Motor to Extrusion Adaptor_v5 (Autodesk Fusion 360 design; units mm, degrees)
Autodesk Fusion 360 part; units mm, degrees
sketch "Sketch1" plane through (0, 0, 0) normal (0, 0, 1) x (1, 0, 0)
  line L0 (0, 0) -> (84, 0)
  line L1 (84, 0) -> (84, 60)
  line L2 (84, 60) -> (0, 60)
  line L3 (0, 60) -> (0, 0)
  line L4 (5, 60) -> (5, 0) construction
  line L5 (79, 60) -> (79, 0) construction
  line L6 (5, 50) -> (79, 50) construction
  line L7 (5, 10) -> (79, 10) construction
  line L8 (7.75, 50) -> (7.75, 10) construction
  line L9 (76.25, 50) -> (76.25, 10) construction
  line L10 (5, 55) -> (79, 55) construction
  line L11 (5, 5) -> (79, 5) construction
  line L12 (7.75, 10) -> (7.75, 5) construction
  line L13 (7.75, 50) -> (7.75, 55) construction
  line L14 (76.25, 50) -> (76.25, 55) construction
  line L15 (76.25, 10) -> (76.25, 5) construction
  line L16 (7.75, 15) -> (76.25, 15) construction
  line L17 (7.75, 45) -> (76.25, 45) construction
  line L18 (5, 55) -> (5, 45)
  arc A0 (5, 45) -> (10.5, 45) centre (7.75, 45) ccw
  line L19 (10.5, 45) -> (10.5, 55)
  arc A1 (10.5, 55) -> (5, 55) centre (7.75, 55) ccw
  line L20 (7.75, 55) -> (7.75, 45) construction
  line L21 (10.5, 5) -> (10.5, 15)
  arc A2 (10.5, 15) -> (5, 15) centre (7.75, 15) ccw
  line L22 (5, 15) -> (5, 5)
  arc A3 (5, 5) -> (10.5, 5) centre (7.75, 5) ccw
  line L23 (7.75, 5) -> (7.75, 15) construction
  line L24 (73.5, 55) -> (73.5, 45)
  arc A4 (73.5, 45) -> (79, 45) centre (76.25, 45) ccw
  line L25 (79, 45) -> (79, 55)
  arc A5 (79, 55) -> (73.5, 55) centre (76.25, 55) ccw
  line L26 (76.25, 55) -> (76.25, 45) construction
  line L27 (73.5, 15) -> (73.5, 5)
  arc A6 (73.5, 5) -> (79, 5) centre (76.25, 5) ccw
  line L28 (79, 5) -> (79, 15)
  arc A7 (79, 15) -> (73.5, 15) centre (76.25, 15) ccw
  line L29 (76.25, 15) -> (76.25, 5) construction
  line L30 (15.5, 55) -> (68.5, 55)
  line L31 (68.5, 55) -> (68.5, 5)
  line L32 (68.5, 5) -> (15.5, 5)
  line L33 (15.5, 5) -> (15.5, 55)
  line L34 (15.5, 55) -> (68.5, 5) construction
  line L35 (68.5, 55) -> (15.5, 5) construction
  line L36 (68.5, 55) -> (68.5, 5) construction
  line L37 (15.5, 55) -> (15.5, 5) construction
  line L38 (50, 15) -> (50, 45) construction
  line L39 (34, 15) -> (34, 45) construction
  line L40 (31.9215, 18.6) -> (29.8431, 15)
  line L41 (29.8431, 15) -> (31.9215, 11.4)
  line L42 (31.9215, 11.4) -> (36.0785, 11.4)
  line L43 (36.0785, 11.4) -> (38.1569, 15)
  line L44 (38.1569, 15) -> (36.0785, 18.6)
  line L45 (36.0785, 18.6) -> (31.9215, 18.6)
  line L46 (36.0785, 41.4) -> (38.1569, 45)
  line L47 (38.1569, 45) -> (36.0785, 48.6)
  line L48 (36.0785, 48.6) -> (31.9215, 48.6)
  line L49 (31.9215, 48.6) -> (29.8431, 45)
  line L50 (29.8431, 45) -> (31.9215, 41.4)
  line L51 (31.9215, 41.4) -> (36.0785, 41.4)
  line L52 (52.0785, 41.4) -> (54.1569, 45)
  line L53 (54.1569, 45) -> (52.0785, 48.6)
  line L54 (52.0785, 48.6) -> (47.9215, 48.6)
  line L55 (47.9215, 48.6) -> (45.8431, 45)
  line L56 (45.8431, 45) -> (47.9215, 41.4)
  line L57 (47.9215, 41.4) -> (52.0785, 41.4)
  line L58 (47.9215, 18.6) -> (45.8431, 15)
  line L59 (45.8431, 15) -> (47.9215, 11.4)
  line L60 (47.9215, 11.4) -> (52.0785, 11.4)
  line L61 (52.0785, 11.4) -> (54.1569, 15)
  line L62 (54.1569, 15) -> (52.0785, 18.6)
  line L63 (52.0785, 18.6) -> (47.9215, 18.6)
  point P0 (42, 30)
  point P1 (34, 15)
  point P2 (34, 45)
  point P3 (50, 45)
  point P4 (50, 15)
  dimension "d1" = 84
  dimension "d2" = 60
  dimension "d3" = 5
  dimension "d4" = 5
  dimension "d5" = 2.75
  dimension "d6" = 2.75
  dimension "d7" = 40
  dimension "d8" = 5
  dimension "d9" = 5
  dimension "d10" = 5
  dimension "d11" = 5
  dimension "d12" = 5.5
  dimension "d13" = 5.5
  dimension "d16" = 53
  dimension "d17" = 50
  dimension "d18" = 18.5
  dimension "d19" = 18.5
  dimension "d20" = 3.6
  dimension "d21" = 3.6
  dimension "d22" = 3.6
  dimension "d23" = 3.6
  constraint horizontal L0
  constraint vertical L1
  constraint horizontal L2
  constraint vertical L3
  constraint coincident L0.start L3.end
  constraint coincident L2 L4.start
  constraint coincident L0 L4.end
  constraint perpendicular L0 L4
  constraint coincident L2 L5.start
  constraint perpendicular L2 L5
  constraint coincident L4 L6.start
  constraint coincident L5 L6.end
  constraint perpendicular L5 L6
  constraint coincident L4 L7.start
  constraint coincident L5 L7.end
  constraint perpendicular L5 L7
  constraint coincident L6 L8.start
  constraint coincident L7 L8.end
  constraint perpendicular L7 L8
  constraint coincident L6 L9.start
  constraint coincident L7 L9.end
  constraint perpendicular L7 L9
  constraint coincident L4 L10.start
  constraint coincident L5 L10.end
  constraint perpendicular L5 L10
  constraint coincident L4 L11.start
  constraint coincident L5 L11.end
  constraint perpendicular L5 L11
  constraint coincident L11 L12.end
  constraint perpendicular L11 L12
  constraint coincident L10 L13.end
  constraint perpendicular L10 L13
  constraint coincident L10 L14.end
  constraint perpendicular L10 L14
  constraint coincident L11 L15.end
  constraint perpendicular L11 L15
  constraint coincident L8 L16.start
  constraint coincident L9 L16.end
  constraint perpendicular L9 L16
  constraint coincident L8 L17.start
  constraint perpendicular L8 L17
  constraint tangent L18 A0
  constraint tangent A0 L19
  constraint parallel L18 L19
  constraint tangent L19 A1
  constraint tangent L18 A1
  constraint coincident L17.start A0.centre
  constraint perpendicular L17 L20
  constraint coincident L13.end A1.centre
  constraint tangent L21 A2
  constraint tangent A2 L22
  constraint parallel L21 L22
  constraint tangent L22 A3
  constraint tangent L21 A3
  constraint coincident L16.start A2.centre
  constraint perpendicular L16 L23
  constraint coincident L12.end A3.centre
  constraint tangent L24 A4
  constraint tangent A4 L25
  constraint parallel L24 L25
  constraint tangent L25 A5
  constraint tangent L24 A5
  constraint coincident L17.end A4.centre
  constraint perpendicular L17 L26
  constraint coincident L14.end A5.centre
  constraint tangent L27 A6
  constraint tangent A6 L28
  constraint parallel L27 L28
  constraint tangent L28 A7
  constraint tangent L27 A7
  constraint coincident L15.end A6.centre
  constraint perpendicular L11 L29
  constraint coincident L16.end A7.centre
  constraint horizontal L30
  constraint perpendicular L30 L31
  constraint parallel L30 L32
  constraint parallel L31 L33
  constraint coincident L34 P0
  constraint coincident L35 P0
  constraint coincident L16 P4
  constraint coincident L17 P3
  constraint perpendicular L17 L38
  constraint coincident L16 P1
  constraint coincident L17 P2
  constraint perpendicular L17 L39
  constraint coincident P1 L39.start
  constraint coincident P2 L39.end
  constraint coincident P3 L38.end
  constraint coincident P4 L38.start
  measures "d1" distance of L0.start L0.end
  measures "d2" distance of L0.start L2.end
  measures "d3" distance of L3 L4
  measures "d4" distance of L1 L5
  measures "d5" distance of L4 L8
  measures "d6" distance of L5 L9
  measures "d7" distance of L6 L7
  measures "d8" distance of L6 L10
  measures "d9" distance of L6 L17
  measures "d10" distance of L7 L16
  measures "d11" distance of L7 L11
  measures "d12" diameter of A0
  measures "d13" diameter of A2
  measures "d16" distance of L31.end L32.end
  measures "d17" distance of L30.end L31.end
  measures "d18" distance of L37 L39
  measures "d19" distance of L31 L38
  measures "d20" distance of P1 L45
  measures "d21" distance of P2 L51
  measures "d22" distance of P3 L57
  measures "d23" distance of P4 L63
extrude "Extrude1" add sketch "Sketch1" against normal blind 5.3 contours L0 L1 L2 L3 | L30 L31 L32 L33
extrude "Extrude2" add sketch "Sketch1" along normal blind 0.2 contours L30 L31 L32 L33 | L40 L41 L42 L43 L44 L45 | L46 L47 L48 L49 L50 L51 | L52 L53 L54 L55 L56 L57 | L58 L59 L60 L61 L62 L63
sketch "Sketch2" plane through (0, 0, 0.2) normal (0, 0, 1) x (-1, 0, 0)
  line L0 (-15.5, -5) -> (-68.5, -5)
  line L1 (-68.5, -5) -> (-68.5, -55)
  line L2 (-68.5, -55) -> (-15.5, -55)
  line L3 (-15.5, -55) -> (-15.5, -5)
  circle A0 centre (-34, -45) radius 2.1
  circle A1 centre (-50, -45) radius 2.1
  circle A2 centre (-34, -15) radius 2.1
  circle A3 centre (-50, -15) radius 2.1
  point P0 (-50, -45)
  point P1 (-34, -45)
  point P2 (-34, -15)
  point P3 (-50, -15)
  dimension "d26" = 4.2
  dimension "d27" = 4.2
  dimension "d28" = 4.2
  dimension "d29" = 4.2
  constraint coincident P1 A0.centre
  constraint coincident P0 A1.centre
  constraint coincident P2 A2.centre
  constraint coincident P3 A3.centre
  measures "d26" diameter of A0
  measures "d28" diameter of A2
extrude "Extrude3" add sketch "Sketch2" along normal blind 3.5
